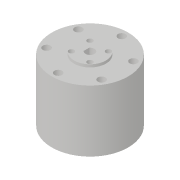
# Autodesk Inventor part: wheel insert
Saved by Autodesk Inventor 2018 (Build 220112000, 112)
## iProperties
Created: 2019-09-21
Part Number: wheel insert
Material: Generic
Document SubType Name: Modeling
Designer: ball
Density: 1 g/cm^3
Appearance: Default
Author: ball
Autodesk Inventor part; units mm, degrees
ref_plane "YZ Plane" through (0, 0, 0) normal (1, 0, 0) x (0, 1, 0)
ref_plane "XZ Plane" through (0, 0, 0) normal (0, 1, 0) x (-1, 0, 0)
ref_plane "XY Plane" through (0, 0, 0) normal (0, 0, 1) x (1, 0, 0)
sketch "Sketch1" plane through (0, 0, 0) normal (0, 1, 0) x (-1, 0, 0)
  circle A0 centre (144.9959, -68.2625) radius 28.4988
  arc A1 (147.6375, -66.2393) -> (147.6375, -70.2857) centre (144.9959, -68.2625) ccw
  line L0 (147.6375, -70.2857) -> (147.6375, -66.2393)
  circle A2 centre (144.9959, -92.0115) radius 2.794
  circle A3 centre (144.9959, -44.5135) radius 2.794
  circle A4 centre (165.5631, -80.137) radius 2.794
  circle A5 centre (124.4287, -56.388) radius 2.794
  circle A6 centre (165.5631, -56.388) radius 2.794
  circle A7 centre (124.4287, -80.137) radius 2.794
  circle A8 centre (144.9959, -44.5135) radius 2.794
  circle A9 centre (144.9959, -92.0115) radius 2.794
  circle A10 centre (124.4287, -56.388) radius 2.794
  circle A11 centre (165.5631, -80.137) radius 2.794
  circle A12 centre (124.4287, -80.137) radius 2.794
  circle A13 centre (165.5631, -56.388) radius 2.794
  circle A14 centre (151.9123, -75.1789) radius 1.9685
  circle A15 centre (151.9123, -61.3461) radius 1.9685
  circle A16 centre (138.0795, -61.3461) radius 1.9685
  circle A17 centre (138.0795, -75.1789) radius 1.9685
  point P0 (0, 0)
  dimension "d1" = 6.6548
  dimension "d2" = 5.969
  dimension "d3" = 5.588
  dimension "d4" = 23.749
  dimension "d7" = 360
  dimension "d9" = 3.937
  dimension "d14" = 360
  constraints: 18 centre point, 2 end point, 2 point on circle, 1 coincident, 1 vertical, 34 other
  measures "d1" diameter of A1
  measures "d3" diameter of A2
  measures "d4" distance of A0.centre A2.centre
  measures "d9" diameter of A14
extrude "Extrusion1" add sketch "Sketch1" along normal blind 50.038
sketch "Sketch2" plane through (-144.9959, 50.038, -68.2625) normal (0, 1, 0) x (1, 0, 0)
  circle A0 centre (0, 0) radius 11.8872
  circle A1 centre (0, 0) radius 28.4988
  point P0 (144.9959, -68.2625)
  dimension "d18" = 23.7744
  constraints: 2 centre point, 1 coincident
  measures "d18" diameter of A0
extrude "Extrusion2" cut sketch "Sketch2" against normal blind 2.032
sketch "Sketch3" plane through (-144.9959, 0, -68.2625) normal (0, -1, 0) x (1, 0, 0)
  arc A0 (-2.6416, -2.0232) -> (-2.6416, 2.0232) centre (0, 0) ccw projected
  circle A1 centre (0, 0) radius 11.8872
  circle A2 centre (0, 0) radius 28.4988
  point P0 (144.9959, 68.2625)
  constraints: 2 centre point, 2 coincident
extrude "Extrusion3" cut sketch "Sketch3" against normal blind 2.032
body "Solid1"
